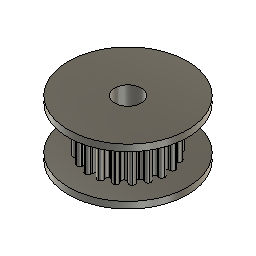
toothed idler pulley, 4mm shaft, 20 teeth v5 (Autodesk Fusion 360 design; units mm, degrees)
Autodesk Fusion 360 part; units mm, degrees
sketch "Sketch1" plane through (0, 0, 0) normal (0, 0, 1) x (1, 0, 0) in component "idler pulley"
  circle A0 centre (-19.8485, 10.6997) radius 9
  circle A1 centre (-19.8485, 10.6997) radius 2
  line L0 (-19.8485, 10.6997) -> (-14.5702, 12.4148) construction
  line L1 (-19.8485, 10.6997) -> (-14.7985, 10.6997) construction
  line L2 (-19.8485, 10.6997) -> (-14.8607, 11.4897) construction
  line L3 (-14.8275, 11.0683) -> (-14.8317, 11.1211)
  line L4 (-14.4955, 11.5475) -> (-14.3004, 11.5784)
  line L5 (-14.5702, 12.4148) -> (-14.5062, 12.4355)
  line L6 (-14.4288, 10.6997) -> (-14.2985, 10.6997)
  line L7 (-13.974, 12.0669) -> (-13.9936, 12.1485)
  arc A2 (-14.4955, 11.5475) -> (-14.8317, 11.1211) centre (-14.4329, 11.1525) ccw
  arc A3 (-14.8275, 11.0683) -> (-14.4288, 10.6997) centre (-14.4288, 11.0997) ccw
  arc A4 (-13.9936, 12.1485) -> (-14.5062, 12.4355) centre (-14.3826, 12.0551) ccw
  arc A5 (-14.3004, 11.5784) -> (-13.974, 12.0669) centre (-14.363, 11.9735) ccw
  line L8 (-14.694, 12.3745) -> (-14.5702, 12.4148)
  arc A6 (-15.1872, 12.6019) -> (-14.694, 12.3745) centre (-14.8176, 12.7549) ccw
  line L9 (-15.1872, 12.6019) -> (-15.2074, 12.6507)
  arc A7 (-15.0195, 13.1602) -> (-15.2074, 12.6507) centre (-14.8379, 12.8038) ccw
  line L10 (-15.0195, 13.1602) -> (-14.8435, 13.2499)
  arc A8 (-14.8435, 13.2499) -> (-14.684, 13.8153) centre (-15.0251, 13.6063) ccw
  line L11 (-14.684, 13.8153) -> (-14.7279, 13.8869)
  arc A9 (-14.7279, 13.8869) -> (-15.304, 14.0015) centre (-15.0689, 13.6779) ccw
  line L12 (-15.3585, 13.9619) -> (-15.304, 14.0015)
  line L13 (-15.4638, 13.8854) -> (-15.3585, 13.9619)
  arc A10 (-16.0031, 13.9492) -> (-15.4638, 13.8854) centre (-15.699, 14.209) ccw
  line L14 (-16.0031, 13.9492) -> (-16.0375, 13.9894)
  arc A11 (-16.0162, 14.5321) -> (-16.0375, 13.9894) centre (-15.7333, 14.2492) ccw
  line L15 (-16.0162, 14.5321) -> (-15.8765, 14.6717)
  arc A12 (-15.8765, 14.6717) -> (-15.8996, 15.2587) centre (-16.1593, 14.9546) ccw
  line L16 (-15.8996, 15.2587) -> (-15.9634, 15.3132)
  arc A13 (-15.9634, 15.3132) -> (-16.5468, 15.2442) centre (-16.2232, 15.0091) ccw
  line L17 (-16.5863, 15.1898) -> (-16.5468, 15.2442)
  line L18 (-16.6629, 15.0844) -> (-16.5863, 15.1898)
  arc A14 (-17.1955, 14.9784) -> (-16.6629, 15.0844) centre (-16.9865, 15.3195) ccw
  line L19 (-17.1955, 14.9784) -> (-17.2406, 15.0061)
  arc A15 (-17.388, 15.5287) -> (-17.2406, 15.0061) centre (-17.0316, 15.3471) ccw
  line L20 (-17.388, 15.5287) -> (-17.2983, 15.7047)
  arc A16 (-17.2983, 15.7047) -> (-17.5017, 16.2559) centre (-17.6547, 15.8863) ccw
  line L21 (-17.5017, 16.2559) -> (-17.5792, 16.288)
  arc A17 (-17.5792, 16.288) -> (-18.1127, 16.0421) centre (-17.7323, 15.9185) ccw
  line L22 (-18.1335, 15.9781) -> (-18.1127, 16.0421)
  line L23 (-18.1737, 15.8542) -> (-18.1335, 15.9781)
  arc A18 (-18.6475, 15.5889) -> (-18.1737, 15.8542) centre (-18.5541, 15.9778) ccw
  line L24 (-18.6475, 15.5889) -> (-18.699, 15.6012)
  arc A19 (-19.0007, 16.0527) -> (-18.699, 15.6012) centre (-18.6056, 15.9902) ccw
  line L25 (-19.0007, 16.0527) -> (-18.9698, 16.2478)
  arc A20 (-18.9698, 16.2478) -> (-19.3335, 16.7092) centre (-19.3649, 16.3104) ccw
  line L26 (-19.3335, 16.7092) -> (-19.4171, 16.7158)
  arc A21 (-19.4171, 16.7158) -> (-19.8485, 16.317) centre (-19.4485, 16.317) ccw
  line L27 (-19.8485, 16.2497) -> (-19.8485, 16.317)
  line L28 (-19.8485, 16.1195) -> (-19.8485, 16.2497)
  arc A22 (-20.2171, 15.7207) -> (-19.8485, 16.1195) centre (-20.2485, 16.1195) ccw
  line L29 (-20.2171, 15.7207) -> (-20.2699, 15.7165)
  arc A23 (-20.6964, 16.0527) -> (-20.2699, 15.7165) centre (-20.3013, 16.1153) ccw
  line L30 (-20.6964, 16.0527) -> (-20.7273, 16.2478)
  arc A24 (-20.7273, 16.2478) -> (-21.2157, 16.5742) centre (-21.1223, 16.1853) ccw
  line L31 (-21.2157, 16.5742) -> (-21.2973, 16.5546)
  arc A25 (-21.2973, 16.5546) -> (-21.5844, 16.0421) centre (-21.2039, 16.1657) ccw
  line L32 (-21.5636, 15.9781) -> (-21.5844, 16.0421)
  line L33 (-21.5233, 15.8542) -> (-21.5636, 15.9781)
  arc A26 (-21.7507, 15.361) -> (-21.5233, 15.8542) centre (-21.9037, 15.7306) ccw
  line L34 (-21.7507, 15.361) -> (-21.7996, 15.3408)
  arc A27 (-22.309, 15.5287) -> (-21.7996, 15.3408) centre (-21.9526, 15.7103) ccw
  line L35 (-22.309, 15.5287) -> (-22.3987, 15.7047)
  arc A28 (-22.3987, 15.7047) -> (-22.9641, 15.8642) centre (-22.7551, 15.5231) ccw
  line L36 (-22.9641, 15.8642) -> (-23.0357, 15.8204)
  arc A29 (-23.0357, 15.8204) -> (-23.1503, 15.2442) centre (-22.8267, 15.4793) ccw
  line L37 (-23.1107, 15.1898) -> (-23.1503, 15.2442)
  line L38 (-23.0342, 15.0844) -> (-23.1107, 15.1898)
  arc A30 (-23.098, 14.5451) -> (-23.0342, 15.0844) centre (-23.3578, 14.8493) ccw
  line L39 (-23.098, 14.5451) -> (-23.1382, 14.5107)
  arc A31 (-23.6809, 14.5321) -> (-23.1382, 14.5107) centre (-23.398, 14.8149) ccw
  line L40 (-23.6809, 14.5321) -> (-23.8205, 14.6717)
  arc A32 (-23.8205, 14.6717) -> (-24.4075, 14.6487) centre (-24.1034, 14.3889) ccw
  line L41 (-24.4075, 14.6487) -> (-24.462, 14.5848)
  arc A33 (-24.462, 14.5848) -> (-24.393, 14.0015) centre (-24.1579, 14.3251) ccw
  line L42 (-24.3386, 13.9619) -> (-24.393, 14.0015)
  line L43 (-24.2332, 13.8854) -> (-24.3386, 13.9619)
  arc A34 (-24.1272, 13.3528) -> (-24.2332, 13.8854) centre (-24.4683, 13.5618) ccw
  line L44 (-24.1272, 13.3528) -> (-24.1549, 13.3076)
  arc A35 (-24.6776, 13.1602) -> (-24.1549, 13.3076) centre (-24.496, 13.5166) ccw
  line L45 (-24.6776, 13.1602) -> (-24.8536, 13.2499)
  arc A36 (-24.8536, 13.2499) -> (-25.4047, 13.0466) centre (-25.0351, 12.8935) ccw
  line L46 (-25.4047, 13.0466) -> (-25.4368, 12.969)
  arc A37 (-25.4368, 12.969) -> (-25.1909, 12.4355) centre (-25.0673, 12.816) ccw
  line L47 (-25.1269, 12.4148) -> (-25.1909, 12.4355)
  line L48 (-25.003, 12.3745) -> (-25.1269, 12.4148)
  arc A38 (-24.7377, 11.9007) -> (-25.003, 12.3745) centre (-25.1266, 11.9941) ccw
  line L49 (-24.7377, 11.9007) -> (-24.75, 11.8492)
  arc A39 (-25.2015, 11.5475) -> (-24.75, 11.8492) centre (-25.139, 11.9426) ccw
  line L50 (-25.2015, 11.5475) -> (-25.3966, 11.5784)
  arc A40 (-25.3966, 11.5784) -> (-25.858, 11.2148) centre (-25.4592, 11.1834) ccw
  line L51 (-25.858, 11.2148) -> (-25.8646, 11.1311)
  arc A41 (-25.8646, 11.1311) -> (-25.4658, 10.6997) centre (-25.4658, 11.0997) ccw
  line L52 (-25.3985, 10.6997) -> (-25.4658, 10.6997)
  line L53 (-25.2683, 10.6997) -> (-25.3985, 10.6997)
  arc A42 (-24.8695, 10.3311) -> (-25.2683, 10.6997) centre (-25.2683, 10.2997) ccw
  line L54 (-24.8695, 10.3311) -> (-24.8654, 10.2783)
  arc A43 (-25.2015, 9.8519) -> (-24.8654, 10.2783) centre (-25.2641, 10.2469) ccw
  line L55 (-25.2015, 9.8519) -> (-25.3966, 9.821)
  arc A44 (-25.3966, 9.821) -> (-25.723, 9.3325) centre (-25.3341, 9.4259) ccw
  line L56 (-25.723, 9.3325) -> (-25.7034, 9.2509)
  arc A45 (-25.7034, 9.2509) -> (-25.1909, 8.9639) centre (-25.3145, 9.3443) ccw
  line L57 (-25.1269, 8.9847) -> (-25.1909, 8.9639)
  line L58 (-25.003, 9.0249) -> (-25.1269, 8.9847)
  arc A46 (-24.5099, 8.7976) -> (-25.003, 9.0249) centre (-24.8794, 8.6445) ccw
  line L59 (-24.5099, 8.7976) -> (-24.4896, 8.7487)
  arc A47 (-24.6776, 8.2392) -> (-24.4896, 8.7487) centre (-24.8592, 8.5956) ccw
  line L60 (-24.6776, 8.2392) -> (-24.8536, 8.1495)
  arc A48 (-24.8536, 8.1495) -> (-25.013, 7.5841) centre (-24.672, 7.7931) ccw
  line L61 (-25.013, 7.5841) -> (-24.9692, 7.5126)
  arc A49 (-24.9692, 7.5126) -> (-24.393, 7.398) centre (-24.6281, 7.7216) ccw
  line L62 (-24.3386, 7.4375) -> (-24.393, 7.398)
  line L63 (-24.2332, 7.5141) -> (-24.3386, 7.4375)
  arc A50 (-23.6939, 7.4502) -> (-24.2332, 7.5141) centre (-23.9981, 7.1904) ccw
  line L64 (-23.6939, 7.4502) -> (-23.6595, 7.41)
  arc A51 (-23.6809, 6.8674) -> (-23.6595, 7.41) centre (-23.9637, 7.1502) ccw
  line L65 (-23.6809, 6.8674) -> (-23.8205, 6.7277)
  arc A52 (-23.8205, 6.7277) -> (-23.7975, 6.1407) centre (-23.5377, 6.4448) ccw
  line L66 (-23.7975, 6.1407) -> (-23.7337, 6.0862)
  arc A53 (-23.7337, 6.0862) -> (-23.1503, 6.1552) centre (-23.4739, 6.3903) ccw
  line L67 (-23.1107, 6.2097) -> (-23.1503, 6.1552)
  line L68 (-23.0342, 6.315) -> (-23.1107, 6.2097)
  arc A54 (-22.5016, 6.421) -> (-23.0342, 6.315) centre (-22.7106, 6.0799) ccw
  line L69 (-22.5016, 6.421) -> (-22.4564, 6.3933)
  arc A55 (-22.309, 5.8707) -> (-22.4564, 6.3933) centre (-22.6654, 6.0523) ccw
  line L70 (-22.309, 5.8707) -> (-22.3987, 5.6947)
  arc A56 (-22.3987, 5.6947) -> (-22.1954, 5.1435) centre (-22.0423, 5.5131) ccw
  line L71 (-22.1954, 5.1435) -> (-22.1178, 5.1114)
  arc A57 (-22.1178, 5.1114) -> (-21.5844, 5.3574) centre (-21.9648, 5.481) ccw
  line L72 (-21.5636, 5.4213) -> (-21.5844, 5.3574)
  line L73 (-21.5233, 5.5452) -> (-21.5636, 5.4213)
  arc A58 (-21.0495, 5.8106) -> (-21.5233, 5.5452) centre (-21.1429, 5.4216) ccw
  line L74 (-21.0495, 5.8106) -> (-20.9981, 5.7982)
  arc A59 (-20.6964, 5.3467) -> (-20.9981, 5.7982) centre (-21.0914, 5.4092) ccw
  line L75 (-20.6964, 5.3467) -> (-20.7273, 5.1516)
  arc A60 (-20.7273, 5.1516) -> (-20.3636, 4.6902) centre (-20.3322, 5.089) ccw
  line L76 (-20.3636, 4.6902) -> (-20.2799, 4.6837)
  arc A61 (-20.2799, 4.6837) -> (-19.8485, 5.0824) centre (-20.2485, 5.0824) ccw
  line L77 (-19.8485, 5.1497) -> (-19.8485, 5.0824)
  line L78 (-19.8485, 5.2799) -> (-19.8485, 5.1497)
  arc A62 (-19.4799, 5.6787) -> (-19.8485, 5.2799) centre (-19.4485, 5.2799) ccw
  line L79 (-19.4799, 5.6787) -> (-19.4271, 5.6829)
  arc A63 (-19.0007, 5.3467) -> (-19.4271, 5.6829) centre (-19.3958, 5.2841) ccw
  line L80 (-19.0007, 5.3467) -> (-18.9698, 5.1516)
  arc A64 (-18.9698, 5.1516) -> (-18.4813, 4.8252) centre (-18.5747, 5.2142) ccw
  line L81 (-18.4813, 4.8252) -> (-18.3997, 4.8448)
  arc A65 (-18.3997, 4.8448) -> (-18.1127, 5.3574) centre (-18.4931, 5.2337) ccw
  line L82 (-18.1335, 5.4213) -> (-18.1127, 5.3574)
  line L83 (-18.1737, 5.5452) -> (-18.1335, 5.4213)
  arc A66 (-17.9464, 6.0384) -> (-18.1737, 5.5452) centre (-17.7933, 5.6688) ccw
  line L84 (-17.9464, 6.0384) -> (-17.8975, 6.0586)
  arc A67 (-17.388, 5.8707) -> (-17.8975, 6.0586) centre (-17.7444, 5.6891) ccw
  line L85 (-17.388, 5.8707) -> (-17.2983, 5.6947)
  arc A68 (-17.2983, 5.6947) -> (-16.7329, 5.5352) centre (-16.9419, 5.8763) ccw
  line L86 (-16.7329, 5.5352) -> (-16.6614, 5.5791)
  arc A69 (-16.6614, 5.5791) -> (-16.5468, 6.1552) centre (-16.8704, 5.9201) ccw
  line L87 (-16.5863, 6.2097) -> (-16.5468, 6.1552)
  line L88 (-16.6629, 6.315) -> (-16.5863, 6.2097)
  arc A70 (-16.599, 6.8543) -> (-16.6629, 6.315) centre (-16.3393, 6.5501) ccw
  line L89 (-16.599, 6.8543) -> (-16.5588, 6.8887)
  arc A71 (-16.0162, 6.8674) -> (-16.5588, 6.8887) centre (-16.299, 6.5845) ccw
  line L90 (-16.0162, 6.8674) -> (-15.8765, 6.7277)
  arc A72 (-15.8765, 6.7277) -> (-15.2895, 6.7508) centre (-15.5937, 7.0105) ccw
  line L91 (-15.2895, 6.7508) -> (-15.235, 6.8146)
  arc A73 (-15.235, 6.8146) -> (-15.304, 7.398) centre (-15.5392, 7.0743) ccw
  line L92 (-15.3585, 7.4375) -> (-15.304, 7.398)
  line L93 (-15.4638, 7.5141) -> (-15.3585, 7.4375)
  arc A74 (-15.5698, 8.0467) -> (-15.4638, 7.5141) centre (-15.2287, 7.8377) ccw
  line L94 (-15.5698, 8.0467) -> (-15.5421, 8.0918)
  arc A75 (-15.0195, 8.2392) -> (-15.5421, 8.0918) centre (-15.2011, 7.8828) ccw
  line L95 (-15.0195, 8.2392) -> (-14.8435, 8.1495)
  arc A76 (-14.8435, 8.1495) -> (-14.2923, 8.3528) centre (-14.6619, 8.5059) ccw
  line L96 (-14.2923, 8.3528) -> (-14.2602, 8.4304)
  arc A77 (-14.2602, 8.4304) -> (-14.5062, 8.9639) centre (-14.6298, 8.5834) ccw
  line L97 (-14.5702, 8.9847) -> (-14.5062, 8.9639)
  line L98 (-14.694, 9.0249) -> (-14.5702, 8.9847)
  arc A78 (-14.9594, 9.4987) -> (-14.694, 9.0249) centre (-14.5704, 9.4053) ccw
  line L99 (-14.9594, 9.4987) -> (-14.947, 9.5502)
  arc A79 (-14.4955, 9.8519) -> (-14.947, 9.5502) centre (-14.5581, 9.4568) ccw
  line L100 (-14.4955, 9.8519) -> (-14.3004, 9.821)
  arc A80 (-14.3004, 9.821) -> (-13.8391, 10.1847) centre (-14.2378, 10.216) ccw
  line L101 (-13.8391, 10.1847) -> (-13.8325, 10.2683)
  arc A81 (-13.8325, 10.2683) -> (-14.2312, 10.6997) centre (-14.2312, 10.2997) ccw
  line L102 (-14.2985, 10.6997) -> (-14.2312, 10.6997)
  dimension "d6_1" = 18
  dimension "d8_1" = 4
  dimension "d1" = 18
  dimension "d3" = 5.05
  dimension "d4" = 9
  dimension "d19" = 5.55
  dimension "d20" = 5.05
  dimension "d22" = 0.5
  dimension "d24" = 0.4
  dimension "d25" = 0.4
  dimension "d26" = 0.4
  dimension "d27" = 0.4
  dimension "d29" = 360
  constraint concentric A0 A1
  constraint horizontal L1
  constraint coincident A0.centre A1.centre
  constraint parallel L2 L4
  constraint parallel L0 L5
  constraint parallel L1 L6
  constraint tangent L4 A2
  constraint tangent L3 A3
  constraint tangent L7 A4
  constraint tangent L4 A5
  constraint tangent L5 A4
  constraint tangent L7 A5
  constraint tangent L3 A2
  constraint tangent L6 A3
  measures "d6_1" diameter of A0
  measures "d8_1" diameter of A1
  measures "d1" angle of L0 L1
  measures "d3" distance of A0.centre L2.end
  measures "d4" angle of L1 L2
  measures "d19" distance of A0.centre L0.end
  measures "d20" distance of A0.centre L1.end
  measures "d22" distance of L1.end L6.end
  measures "d24" radius of A3
  measures "d25" radius of A2
  measures "d26" radius of A5
  measures "d27" radius of A4
extrude "Extrude1" add sketch "Sketch1" along normal mid plane 8.5 contours A0 | L3 L4 L5 L6 L7 A2 A3 A4 A5 L8 A6 L9 A7 L10 A8 L11 A9 L12 L13 A10 L14 A11 L15 A12 L16 A13 L17 L18 A14 L19 A15 L20 A16 L21 A17 L22 L23 A18 L24 A19 L25 A20 L26 A21 L27 L28 A22 L29 A23 L30 A24 L31 A25 L32 L33 A26 L34 A27 L35 A28 L36 A29 L37 L38 A30 L39 A31 L40 A32 L41 A33 L42 L43 A34 L44 A35 L45 A36 L46 A37 L47 L48 A38 L49 A39 L50 A40 L51 A41 L52 L53 A42 L54 A43 L55 A44 L56 A45 L57 L58 A46 L59 A47 L60 A48 L61 A49 L62 L63 A50 L64 A51 L65 A52 L66 A53 L67 L68 A54 L69 A55 L70 A56 L71 A57 L72 L73 A58 L74 A59 L75 A60 L76 A61 L77 L78 A62 L79 A63 L80 A64 L81 A65 L82 L83 A66 L84 A67 L85 A68 L86 A69 L87 L88 A70 L89 A71 L90 A72 L91 A73 L92 L93 A74 L94 A75 L95 A76 L96 A77 L97 L98 A78 L99 A79 L100 A80 L101 A81 L102 in component "idler pulley"
extrude "Extrude2" cut sketch "Sketch1" along normal mid plane 6.5 in component "idler pulley"
component "idler pulley" placed x (1, 0, 0) y (0, 1, 0) z (0, 0, 1) at (0, 0, 0)
equation "d6_1 = flange_diameter_1"
equation "d7_1 = pulley_diameter_1"
equation "d8_1 = shaft_diameter_1"
equation "d9_1 = overall_height_1"
equation "d11_1 = belt_space_1"
equation "shaft_diameter_1 = 4 mm"
equation "flange_diameter_1 = 18 mm"
equation "pulley_diameter_1 = 12.1 mm"
equation "belt_space_1 = 6.5 mm"
equation "overall_height_1 = 8.5 mm"
equation "d1 = ( 360 / number_of_teeth ) * 1 deg"
equation "number_of_teeth = 20"
equation "d3 = pulley_diameter_1 / 2 - 1 mm"
equation "d4 = d1 / 2"
equation "d19 = pulley_diameter_1 / 2 - 0.5 mm"
equation "d20 = pulley_diameter_1 / 2 - 1 mm"
equation "d25 = d24"
equation "d27 = d26"
